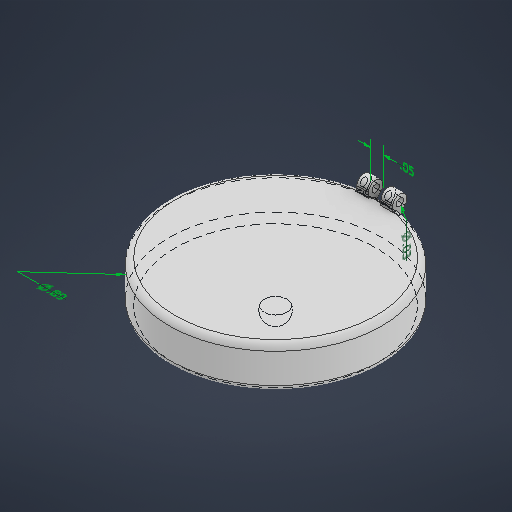
# Autodesk Inventor part: Neck
Saved by Autodesk Inventor 2025.2 (Build 292293000, 293)
## iProperties
Created: 2025-03-31
Part Number: Neck
Material: Generic
Document SubType Name: Modeling
Designer: mylap
Density: 1 g/cm^3
Appearance: Default
Author: mylap
## iProperties of the stored document Neck_3DPrint.ipt
Created: 2025-03-31
Part Number: Neck_3DPrint
Material: Generic
Document SubType Name: Modeling
Designer: mylap
Density: 1 g/cm^3
Appearance: Default
Author: mylap
Autodesk Inventor part; units mm, degrees
ref_plane "XZ Plane" through (0, 0, 0) normal (0, 1, 0) x (-1, 0, 0)
ref_plane "XY Plane" through (0, 0, 0) normal (0, 0, 1) x (1, 0, 0)
sketch "Sketch1" plane through (0, 0, 0) normal (0, 0, 1) x (1, 0, 0)
  line L0 (8.9491, 93.5489) -> (53.3991, 93.5489) construction
  line L1 (53.3991, 93.5489) -> (53.3991, 10.9989) construction
  line L2 (53.3991, 10.9989) -> (8.9491, 10.9989) construction
  line L3 (8.9491, 10.9989) -> (8.9491, 93.5489) construction
  line L4 (42.5105, 69.6145) -> (42.5105, 74.0469)
  line L5 (31.1983, 74.0469) -> (31.1983, 69.6145)
  line L6 (31.1983, 74.0469) -> (42.5105, 74.0469)
  line L7 (42.5105, 69.6145) -> (31.1983, 69.6145)
  circle A0 centre (31.1983, 69.2335) radius 1.27
  line L8 (31.1983, 69.6145) -> (31.1983, 67.9635)
  point P0 (0, 0)
  point P1 (32.4098, 69.6145)
  dimension "d3" = 2.54
  dimension "d4" = 0.381
  constraints: 10 end point, 1 horizontal, 1 parallel, 1 point on line, 1 vertical, 5 other
  measures "d4" distance of L5.end point (31.198, 69.233)
revolve "Revolution1" add sketch "Sketch1" angle 360 about axis through (31.1983, 74.0469, 0) along (0, -1, 0) contours L7 A0 L5 L6 L4 | A0 L8 L7 | L7 L5 A0
fillet "Fillet1" radius 0.635 2 edges at (19.8861, 74.0469, 0) (19.8861, 69.6145, 0)
ref_plane "Work Plane1" through (31.3182, 0, 0) normal (1, 0, 0) x (0, 1, 0)
sketch "Sketch3" plane through (31.3182, 0, 0) normal (1, 0, 0) x (0, 1, 0)
  line L0 (91.7474, 13.6776) -> (91.7474, -13.6861) construction
  line L1 (91.7474, -13.6861) -> (69.2257, -13.6861) construction
  line L2 (69.2257, -13.6861) -> (69.2257, 13.6776) construction
  line L3 (69.2257, 13.6776) -> (91.7474, 13.6776) construction
  circle A0 centre (74.5674, -11.1927) radius 0.765
  circle A1 centre (74.5674, -11.1927) radius 0.3969
  line L4 (74.033, -11.7401) -> (73.4119, -11.3003)
  line L5 (73.4119, -11.3122) -> (73.4119, 11.3122) projected
  line L6 (74.5674, -10.4276) -> (74.0469, -10.4034)
  line L7 (74.0469, 10.6772) -> (74.0469, -10.6772) projected
  line L8 (73.818, -11.0391) -> (73.4119, -11.3003)
  line L9 (74.0727, -10.4046) -> (72.7289, -10.3422)
  line L10 (72.7289, -10.3422) -> (73.4119, -11.3003)
  point P0 (0, 0)
  point P1 (74.0469, -10.632)
  dimension "d49" = 1.53
  dimension "d50" = 0.7937
  constraints: 10 end point, 4 point on line, 3 point on circle, 2 centre point, 1 coincident, 2 other
  measures "d49" diameter of A0
  measures "d50" diameter of A1
extrude "Extrusion1" add sketch "Sketch3" along normal mid plane 3.81 contours A0
extrude "Extrusion2" cut sketch "Sketch3" along normal mid plane 1.3335 contours A0 | A1
extrude "Extrusion3" add sketch "Sketch3" along normal mid plane 3.81 contours A0 L7 L6 | L4 L8 A0 | A0 L8 L5 L9 L7 | L10 L9 L5
extrude "Extrusion4" cut sketch "Sketch3" along normal mid plane 1.3335 contours A0 L7 L6 | L4 L8 A0
body "Solid1"
